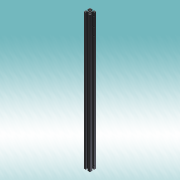
# Autodesk Inventor part: HFSB5-2020-432-LCH-RCH-AH40-BH65
Saved by Autodesk Inventor 2015 (Build 190159000, 159)
## iProperties
Category: PARTsolutions
Company: MISUMI
Created: 2016-03-22
Part Number: HFSB5-2020-432-LCH-RCH-AH40-BH65
Catalog Web Link: www.cadenas.de
Description: NFS5-2020, NFSB5-2020, HFS5-2020, HFSB5-2020, CAF5-2020, HFSY5-2020, NFSF5-2020, HFSF5-2020, HFSFB5-2020, NFST5-2020, HFST5-2020, HFSTB5-2020, HFSH5-2020, HFSC5-2020-HFS5 Series Aluminum Extrusions 20 Square -1 Slot-
Vendor: MISUMI
Document SubType Name: Modeling
Designer: psAdmin
Manufacturer: MISUMI
Mass: 77.6546 g
Surface Area: 750.949 cm^2
Volume: 77.6546 cm^3
Density: 1 g/cm^3
Material: 一般
Appearance: PSOLRGB-175-175-175
PSOL_IDENT_0: {$CADENAS_DATA\23d-libs\misumi\metric\38_al_extrusions_blackets\5\hfs5_2020.prj},608 {VTYP=3D},{NB=H
PSOL_IDENT_1: FSB5-2020-432-LCH-RCH-AH40-BH65},{LINA=HFSB5-2020-432-LCH-RCH-AH40-BH65},{NN=NFS5-2020, NFSB5-2020,
PSOL_IDENT_2: HFS5-2020, HFSB5-2020, CAF5-2020, HFSY5-2020, NFSF5-2020, HFSF5-2020, HFSFB5-2020, NFST5-2020, HFST5
PSOL_IDENT_3: -2020, HFSTB5-2020, HFSH5-2020, HFSC5-2020},{DATE=17.07.2015 10:47:07},{GEOMDATE=28.10.2014 00:00:00
PSOL_IDENT_4: },{VERSION=},{LINEID=140},{LINESUBID=-1},{WBVAR=L,ALT1,ALT2,ALT4,ALT5,CP5,DL5,DR5,ALT6,ALT9,ALT10,AL
PSOL_IDENT_5: T11,HP6,NHL6,DL6,NHR6,DR6,ALT7,ALT8,NH9,AH,BH,CH,DH,EH,NH10,AV,BV,CV,DV,EV,NH11,AP,BP,CP,DP,EP,ALT12
PSOL_IDENT_6: ,ALT13,Z,NH12,XA,XB,XC,XD,XE,NH13,YA,YB,YC,YD,YE,ALT16,HP16,DL16,DR16,ALT17,HQ17,JLP,ALT20}  {NB=HFS
PSOL_IDENT_7: B5-2020-432-LCH-RCH-AH40-BH65},{LINA=HFSB5-2020-432-LCH-RCH-AH40-BH65},{KT=DUMMY},{PN=HFSB5-2020-432
PSOL_IDENT_8: -LCH-RCH-AH40-BH65},{TPS=HFSB5-2020},{MAT=A6N01SS-T5 Aluminum Alloy or 6005A-T5 Aluminum Alloy},{ST=
PSOL_IDENT_9: Black Anodize},{FRMW=20},{FRMH=20},{FRD=4.2},{L=432},{MASS=0.5},{SA=183},{LX=0.742x10^4},{LY=0.742x1
PSOL_IDENT_10: 0^4},{ALT1=},{M1=0},{DPL1=0},{DPR1=0},{ALT1PN=},{ALT2=},{ALT2ALG= '','w/o End Tapping (Heli-Coil Ins
PSOL_IDENT_11: ert)','LHP','with LHP (Tapping on the Left (Heli-Coil Insert))','RHP','with RHP (Tapping on the Righ
PSOL_IDENT_12: t (Heli-Coil Insert))','HPW','with HPW (Tapping on Both Ends (Heli-Coil Insert))' },{M2=0},{DP2=0},{
PSOL_IDENT_13: ALT2PN=},{ALT4=},{ALT4ALG= '', 'w/o SC (High Precision Cut)', 'SC', 'with SC (High Precision Cut)' }
PSOL_IDENT_14: ,{ALT4PN=},{ALT5=},{ALT5ALG= '','w/o 45 Degree Cut','1','with 45 Degree Cut' },{CP5=},{CP5ALG= '','N
PSOL_IDENT_15: /A' },{DL5=},{DL5ALG= '','N/A' },{DR5=},{DR5ALG= '','N/A' },{FRMLALT5=0},{FRMRALT5=0},{ALT5PN=},{ALT
PSOL_IDENT_16: 6=1},{ALT6ALG= '','w/o Fastening Location Wrench Access Hole Alterations','1','with Fastening Locati
PSOL_IDENT_17: on Wrench Access Hole Alterations' },{ALT9=1},{ALT9ALG= '','w/o Location Specified Wrench Access Hol
PSOL_IDENT_18: e Alteratons (Horizontal)','1','with Location Specified Wrench Access Hole Alteratons (Horizontal)'
PSOL_IDENT_19: },{ALT10=},{ALT10ALG= '','w/o Location Specified Wrench Access Hole Alteratons (Vertical)','1','with
PSOL_IDENT_20: Location Specified Wrench Access Hole Alteratons (Vertical)' },{ALT11=},{ALT11ALG= '','w/o Location
PSOL_IDENT_21: Specified Wrench Access Hole Alteratons (Crisscross)','1','with Location Specified Wrench Access Ho
PSOL_IDENT_22: le Alteratons (Crisscross)' },{HP6=LR},{HP6ALG= 'L','Left','R','Right','LR','Both Sides' },{NHL6=C},
PSOL_IDENT_23: {NHL6ALG= 'C','C (Wrench Holes in Single Line)','W','W (Wrench Holes in Two Lines)','E','E (Wrench H
PSOL_IDENT_24: oles in Three Lines)' },{DL6=H},{DL6ALG= 'H','H (Horizontal)','V','V (Vertical)','P','P (Crisscross)'
PSOL_IDENT_25: },{NHR6=C},{NHR6ALG= 'C','C (Wrench Holes in Single Line)','W','W (Wrench Holes in Two Lines)','E','
PSOL_IDENT_26: E (Wrench Holes in Three Lines)' },{DR6=H},{DR6ALG= 'H','H (Horizontal)','V','V (Vertical)','P','P (
PSOL_IDENT_27: Crisscross)' },{HL6=10},{HL6D=10},{HR6=10},{HR6D=10},{J6=20},{J6D=0},{K6=20},{K6D=0},{DD6=7.35},{DD6
PSOL_IDENT_28: ALG=7.35},{ALT7=},{ALT7ALG= '','w/o FL (Shifts The Wrench Hole on The Left Side 3mm Toward The Left
PSOL_IDENT_29: End)','FL','with FL (Shifts The Wrench Hole on The Left Side 3mm Toward The Left End)' },{ALT8=},{AL
PSOL_IDENT_30: T8ALG= '','w/o FR (Shifts The Wrench Hole on The Right Side 3mm Toward The Right End)','FR','with FR
PSOL_IDENT_31: (Shifts The Wrench Hole on The Right Side 3mm Toward The Right End)' },{ALT678PN=-LCH-RCH},{NH9=2},
PSOL_IDENT_32: {NH9MAX=5},{NH9ALG=[1:5/1]},{AH=40.0},{AHMIN=7},{AHMAX=415.5},{AHALG=[7:415.5/0.5]},{BH=65.0},{BHMIN=
PSOL_IDENT_33: 49.5},{BHMAX=425},{BHALG=[49.5:425/0.5]},{CH=0.0},{CHMIN=74.5},{CHMAX=434.5},{CHALG=[0]},{DH=0.0},{D
PSOL_IDENT_34: HMIN=9.5},{DHMAX=444},{DHALG=[0]},{EH=0.0},{EHMIN=9.5},{EHMAX=425},{EHALG=[0]},{NH10=0},{NH10MAX=5},
PSOL_IDENT_35: {NH10ALG=[0]},{AV=0.0},{AVMIN=7},{AVMAX=434.5},{AVALG=[0]},{BV=0.0},{BVMIN=9.5},{BVMAX=444},{BVALG=[
PSOL_IDENT_36: 0]},{CV=0.0},{CVMIN=9.5},{CVMAX=453.5},{CVALG=[0]},{DV=0.0},{DVMIN=9.5},{DVMAX=463},{DVALG=[0]},{EV=
PSOL_IDENT_37: 0.0},{EVMIN=9.5},{EVMAX=425},{EVALG=[0]},{NH11=0},{NH11MAX=5},{NH11ALG=[0]},{AP=0.0},{APMIN=7},{APMA
PSOL_IDENT_38: X=434.5},{APALG=[0]},{BP=0.0},{BPMIN=9.5},{BPMAX=444},{BPALG=[0]},{CP=0.0},{CPMIN=9.5},{CPMAX=453.5}
PSOL_IDENT_39: ,{CPALG=[0]},{DP=0.0},{DPMIN=9.5},{DPMAX=463},{DPALG=[0]},{EP=0.0},{EPMIN=9.5},{EPMAX=425},{EPALG=[0
PSOL_IDENT_40: ]},{ALT9PN=-AH40-BH65},{ALT10PN=},{ALT11PN=},{ALT91011PN=-AH40-BH65},{ALT12=},{ALT12ALG= '','w/o Cou
PSOL_IDENT_41: nterbore Hole in Specified Position (Vertical)','1','with Counterbore Hole in Specified Position (Ve
PSOL_IDENT_42: rtical)' },{ALT13=},{ALT13ALG= '','w/o Counterbore Hole in Specified Position (Horizontal)','1','wit
PSOL_IDENT_43: h Counterbore Hole in Specified Position (Horizontal)' },{Z=},{ZALG= '','N/A' },{DD12=0.0},{DD112=0.
PSOL_IDENT_44: 0},{NH12=0},{NH12MAX=5},{NH12ALG=[0]},{XA=0.0},{XAMIN=7},{XAMAX=427},{XAALG=[0]},{XB=0.0},{XBMIN=2},
PSOL_IDENT_45: {XBMAX=429},{XBALG=[0]},{XC=0.0},{XCMIN=2},{XCMAX=431},{XCALG=[0]},{XD=0.0},{XDMIN=2},{XDMAX=433},{X
PSOL_IDENT_46: DALG=[0]},{XE=0.0},{XEMIN=2},{XEMAX=425},{XEALG=[0]},{NH13=0},{NH13MAX=5},{NH13ALG=[0]},{YA=0.0},{YA
PSOL_IDENT_47: MIN=7},{YAMAX=427},{YAALG=[0]},{YB=0.0},{YBMIN=2},{YBMAX=429},{YBALG=[0]},{YC=0.0},{YCMIN=2},{YCMAX=
PSOL_IDENT_48: 431},{YCALG=[0]},{YD=0.0},{YDMIN=2},{YDMAX=433},{YDALG=[0]},{YE=0.0},{YEMIN=2},{YEMAX=425},{YEALG=[0
PSOL_IDENT_49: ]},{ALT12PN=},{ALT13PN=},{ALT1213PN=},{ALT16=},{ALT16ALG= '','w/o M Type Hole Alteration','1','with
PSOL_IDENT_50: M Type Hole Alteration' },{HP16=},{HP16ALG= '','N/A' },{DL16=},{DL16ALG= '','N/A' },{DR16=},{DR16ALG=
PSOL_IDENT_51: '','N/A' },{H116=0},{D16=0.0},{ALT16PN=},{ALT17=},{ALT17ALG= '','w/o L Type Hole Alteration (Top)','
PSOL_IDENT_52: 1','with L Type Hole Alteration (Top)' },{HQ17=0},{HQ17ALG=0},{JLP=0},{JLPMIN=4.9},{JLPMAX=0},{JLPAL
PSOL_IDENT_53: G=[0]},{L17=0},{D17=0.0},{ALT17PN=},{ALT20=},{ALT20PN=},{ERRORALT01=OK},{ERRORALT02=OK},{ERRORALT05=
PSOL_IDENT_54: OK},{ERRORALT06091=OK},{ERRORALT06092=OK},{ERRORALT06093=OK},{ERRORALT06094=OK},{ERRORALT06101=OK},{
PSOL_IDENT_55: ERRORALT06102=OK},{ERRORALT06103=OK},{ERRORALT06104=OK},{ERRORALT06111=OK},{ERRORALT06112=OK},{ERROR
PSOL_IDENT_56: ALT06113=OK},{ERRORALT06114=OK},{ERRORALT06121=OK},{ERRORALT06122=OK},{ERRORALT06123=OK},{ERRORALT06
PSOL_IDENT_57: 124=OK},{ERRORALT06131=OK},{ERRORALT06132=OK},{ERRORALT06133=OK},{ERRORALT06134=OK},{ERRORALT0616=OK
PSOL_IDENT_58: },{ERRORALT06171=OK},{ERRORALT06172=OK},{ERRORALT06173=OK},{ERRORALT0911=OK},{ERRORALT0913=OK},{ERRO
PSOL_IDENT_59: RALT0916=OK},{ERRORALT0917=OK},{ERRORALT1011=OK},{ERRORALT1012=OK},{ERRORALT1016=OK},{ERRORALT1017=O
PSOL_IDENT_60: K},{ERRORALT1112=OK},{ERRORALT1113=OK},{ERRORALT1116=OK},{ERRORALT1117=OK},{ERRORALT1216=OK},{ERRORA
PSOL_IDENT_61: LT1217=OK},{ERRORALT1316=OK},{ERRORALT1317=OK},{ERRORALT1617=OK},{ERRORPN=},{TFW=0}
NN: NFS5-2020, NFSB5-2020, HFS5-2020, HFSB5-2020, CAF5-2020, HFSY5-2020, NFSF5-2020, HFSF5-2020, HFSFB5-2020, NFST5-2020, HFST5-2020, HFSTB5-2020, HFSH5-2020, HFSC5-2020
NT: HFS5 Series Aluminum Extrusions 20 Square -1 Slot-
NB: HFSB5-2020-432-LCH-RCH-AH40-BH65
NBSYN: $PN.
LINA: HFSB5-2020-432-LCH-RCH-AH40-BH65
PN: HFSB5-2020-432-LCH-RCH-AH40-BH65
TPS: HFSB5-2020
MAT: A6N01SS-T5 Aluminum Alloy or 6005A-T5 Aluminum Alloy
ST: Black Anodize
L: 432
MASS: 0.5
SA: 183
LX: 0.742x10^4
LY: 0.742x10^4
ALT1: w/o End Tapping
M1: 0
DPL1: 0
DPR1: 0
ALT2: w/o End Tapping (Heli-Coil Insert)
M2: 0
DP2: 0
ALT4: w/o SC (High Precision Cut)
ALT5: w/o 45 Degree Cut
CP5: N/A
DL5: N/A
DR5: N/A
ALT6: with Fastening Location Wrench Access Hole Alterations
ALT9: with Location Specified Wrench Access Hole Alteratons (Horizontal)
ALT10: w/o Location Specified Wrench Access Hole Alteratons (Vertical)
ALT11: w/o Location Specified Wrench Access Hole Alteratons (Crisscross)
HP6: Both Sides
NHL6: C (Wrench Holes in Single Line)
DL6: H (Horizontal)
NHR6: C (Wrench Holes in Single Line)
DR6: H (Horizontal)
HL6D: 10
HR6D: 10
J6D: 0
K6D: 0
DD6: 7.35
ALT7: w/o FL (Shifts The Wrench Hole on The Left Side 3mm Toward The Left End)
ALT8: w/o FR (Shifts The Wrench Hole on The Right Side 3mm Toward The Right End)
NH9: 2
AH: 40.0
BH: 65.0
CH: 0.0
DH: 0.0
EH: 0.0
NH10: 0
AV: 0.0
BV: 0.0
CV: 0.0
DV: 0.0
EV: 0.0
NH11: 0
AP: 0.0
BP: 0.0
CP: 0.0
DP: 0.0
EP: 0.0
ALT12: w/o Counterbore Hole in Specified Position (Vertical)
ALT13: w/o Counterbore Hole in Specified Position (Horizontal)
Z: N/A
DD12: 0.0
DD112: 0.0
NH12: 0
XA: 0.0
XB: 0.0
XC: 0.0
XD: 0.0
XE: 0.0
NH13: 0
YA: 0.0
YB: 0.0
YC: 0.0
YD: 0.0
YE: 0.0
ALT16: w/o M Type Hole Alteration
HP16: N/A
DL16: N/A
DR16: N/A
H116: 0
D16: 0.0
ALT17: w/o L Type Hole Alteration (Top)
HQ17: 0
JLP: 0
D17: 0.0
ALT20: w/o CW (End Face C Chamfering)
SUPPLIER: MISUMI
ARTICLENO: HFSB5-2020-432-LCH-RCH-AH40-BH65
BOMINFO: HFSB5-2020-432-LCH-RCH-AH40-BH65
CREATOR: CADENAS GmbH
Title: HFSB5-2020-432-LCH-RCH-AH40-BH65
Author: Cadenas PARTsolutions
Comments: HFS5 Series Aluminum Extrusions 20 Square -1 Slot-
Autodesk Inventor part; units mm, degrees
sketch "Sketch_1" plane through (0, 0, 0) normal (0, 0, 1) x (1, 0, 0)
  line L0 (-10, 3) -> (-8, 3)
  line L1 (-8, 3) -> (-8, 6)
  line L2 (-8, 6) -> (-7.0607, 6)
  line L3 (-7.0607, 6) -> (-4, 2.9393)
  line L4 (-4, 2.9393) -> (-4, 0.5196)
  line L5 (-4, 0.5196) -> (-3.7, 0)
  line L6 (-3.7, 0) -> (-4, -0.5196)
  line L7 (-4, -0.5196) -> (-4, -2.9393)
  line L8 (-4, -2.9393) -> (-7.0607, -6)
  line L9 (-7.0607, -6) -> (-8, -6)
  line L10 (-8, -6) -> (-8, -3)
  line L11 (-8, -3) -> (-10, -3)
  line L12 (-10, -3) -> (-10, -9)
  arc A0 (-10, -9) -> (-9, -10) centre (-9, -9) ccw
  line L13 (-9, -10) -> (-3, -10)
  line L14 (-3, -10) -> (-3, -8)
  line L15 (-3, -8) -> (-6, -8)
  line L16 (-6, -8) -> (-6, -7.0607)
  line L17 (-6, -7.0607) -> (-2.9393, -4)
  line L18 (-2.9393, -4) -> (-0.5196, -4)
  line L19 (-0.5196, -4) -> (0, -3.7)
  line L20 (0, -3.7) -> (0.5196, -4)
  line L21 (0.5196, -4) -> (2.9393, -4)
  line L22 (2.9393, -4) -> (6, -7.0607)
  line L23 (6, -7.0607) -> (6, -8)
  line L24 (6, -8) -> (3, -8)
  line L25 (3, -8) -> (3, -10)
  line L26 (3, -10) -> (9, -10)
  arc A1 (9, -10) -> (10, -9) centre (9, -9) ccw
  line L27 (10, -9) -> (10, -3)
  line L28 (10, -3) -> (8, -3)
  line L29 (8, -3) -> (8, -6)
  line L30 (8, -6) -> (7.0607, -6)
  line L31 (7.0607, -6) -> (4, -2.9393)
  line L32 (4, -2.9393) -> (4, -0.5196)
  line L33 (4, -0.5196) -> (3.7, 0)
  line L34 (3.7, 0) -> (4, 0.5196)
  line L35 (4, 0.5196) -> (4, 2.9393)
  line L36 (4, 2.9393) -> (7.0607, 6)
  line L37 (7.0607, 6) -> (8, 6)
  line L38 (8, 6) -> (8, 3)
  line L39 (8, 3) -> (10, 3)
  line L40 (10, 3) -> (10, 9)
  arc A2 (10, 9) -> (9, 10) centre (9, 9) ccw
  line L41 (9, 10) -> (3, 10)
  line L42 (3, 10) -> (3, 8)
  line L43 (3, 8) -> (6, 8)
  line L44 (6, 8) -> (6, 7.0607)
  line L45 (6, 7.0607) -> (2.9393, 4)
  line L46 (2.9393, 4) -> (0.5196, 4)
  line L47 (0.5196, 4) -> (0, 3.7)
  line L48 (0, 3.7) -> (-0.5196, 4)
  line L49 (-0.5196, 4) -> (-2.9393, 4)
  line L50 (-2.9393, 4) -> (-6, 7.0607)
  line L51 (-6, 7.0607) -> (-6, 8)
  line L52 (-6, 8) -> (-3, 8)
  line L53 (-3, 8) -> (-3, 10)
  line L54 (-3, 10) -> (-9, 10)
  arc A3 (-9, 10) -> (-10, 9) centre (-9, 9) ccw
  line L55 (-10, 9) -> (-10, 3)
  constraints: 112 end point, 8 point on circle, 4 centre point
extrude "Extrusion1" add sketch "Sketch_1" against normal blind 432
sketch "Sketch2" plane through (0, 0, -432) normal (0, 0, -1) x (-1, 0, 0)
  point P0 (0, 0)
hole "Hole1" at (0, 0, -432) direction (0, 0, 1) diameter 4.2 depth 432
sketch "Sketch_13" plane through (0, 0, 0) normal (0, 1, 0) x (1, 0, 0)
  line L0 (10, 10) -> (-10, 10)
  line L1 (-10, 10) -> (-10, 13.675)
  line L2 (-10, 13.675) -> (10, 13.675)
  line L3 (10, 13.675) -> (10, 10)
  line L4 (10, 10) -> (-10, 10)
  constraints: 10 end point
revolve "Revolution1" cut sketch "Sketch_13" angle 360 about axis through (10, 0, -10) along (1, 0, 0)
sketch "Sketch_16" plane through (0, 0, 0) normal (0, 1, 0) x (1, 0, 0)
  line L0 (10, 422) -> (-10, 422)
  line L1 (-10, 422) -> (-10, 425.675)
  line L2 (-10, 425.675) -> (10, 425.675)
  line L3 (10, 425.675) -> (10, 422)
  line L4 (10, 422) -> (-10, 422)
  constraints: 10 end point
revolve "Revolution2" cut sketch "Sketch_16" angle 360 about axis through (10, 0, -422) along (1, 0, 0)
sketch "Sketch_62" plane through (0, 0, 0) normal (0, 1, 0) x (1, 0, 0)
  line L0 (10, 40) -> (-10, 40)
  line L1 (-10, 40) -> (-10, 43.675)
  line L2 (-10, 43.675) -> (10, 43.675)
  line L3 (10, 43.675) -> (10, 40)
  line L4 (10, 40) -> (-10, 40)
  constraints: 10 end point
revolve "Revolution3" cut sketch "Sketch_62" angle 360 about axis through (10, 0, -40) along (1, 0, 0)
sketch "Sketch_25" plane through (0, 0, 0) normal (0, 1, 0) x (1, 0, 0)
  line L0 (10, 65) -> (-10, 65)
  line L1 (-10, 65) -> (-10, 68.675)
  line L2 (-10, 68.675) -> (10, 68.675)
  line L3 (10, 68.675) -> (10, 65)
  line L4 (10, 65) -> (-10, 65)
  constraints: 10 end point
revolve "Revolution4" cut sketch "Sketch_25" angle 360 about axis through (10, 0, -65) along (1, 0, 0)
ref_plane "C1_XY" through (0, 0, 0) normal (0, 0, 1) x (1, 0, 0)
ref_plane "C1_YZ" through (0, 0, 0) normal (1, 0, 0) x (0, 1, 0)
ref_plane "C1_ZX" through (0, 0, 0) normal (0, 1, 0) x (0, 0, 1)
body "Solid1"
